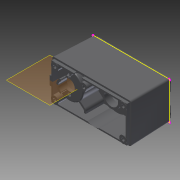
# Autodesk Inventor part: 276-2181-002 Rev1
Saved by Autodesk Inventor 2013 (Build 170138000, 138)
## iProperties
Category: Motors
Company: Autodesk Inc.
Created: 2012-01-21
Part Number: 276-2181-002 Rev1
Material: Generic
Document SubType Name: Modeling
Designer: Autodesk Inc.
Density: 1 g/cm^3
Catalog Web Link: http://www.vexrobotics.com/276-2181.html
Vendor: VEX
Author: Autodesk Inc.
Autodesk Inventor part; units mm, degrees
sketch "Sketch1" plane through (0, 0, 0) normal (0, 0, 1) x (1, 0, 0)
  line L0 (-20, -10) -> (20, -10)
  line L1 (20, -10) -> (20, 10)
  line L2 (-20, 10) -> (20, 10)
  line L3 (-20, -10) -> (-20, 10)
  point P0 (-19.0003, -10)
  point P1 (19.0003, -10)
  point P2 (20, -9.0003)
  point P3 (20, 9.0003)
  point P4 (19.0003, 10)
  point P5 (-19.0003, 10)
  point P6 (-20, 9.0003)
  point P7 (-20, -9.0003)
  constraints: 8 end point, 8 point on line, 1 parallel
extrude "Extrusion1" add sketch "Sketch1" against normal blind 19.9898 draft -1.5
fillet "Fillet3" radius 1.0033 4 edges at (19.7383, 9.7383, -9.9949) (19.7383, -9.7383, -9.9949) (-19.7383, 9.7383, -9.9949) (-19.7383, -9.7383, -9.9949)
sketch "Sketch2" plane through (0, 0, 0) normal (0, 0, 1) x (1, 0, 0)
  arc A0 (-10.02, 6.9107) -> (-9.998, 7.0969) centre (-10.798, 7.0969) ccw
  arc A1 (-10.02, 6.9107) -> (-9.9362, 6.8636) centre (-9.9713, 6.8991) ccw
  arc A2 (-9.0524, 7.5864) -> (-9.9362, 6.8636) centre (-5.7003, 2.586) ccw
  arc A3 (-8.5705, 8.418) -> (-9.0524, 7.5864) centre (-8.188, 7.6409) ccw
  arc A4 (-7.7003, 8.7706) -> (-8.5705, 8.418) centre (-5.7003, 2.586) ccw
  line L0 (-7.7003, 8.7706) -> (-7.7003, 9.2)
  line L1 (-17.3, 9.2) -> (-7.7003, 9.2)
  line L2 (-18.5, 8.5) -> (-9.998, 8.5)
  line L3 (-9.998, 8.5) -> (-9.998, 7.0969)
  line L4 (17.3, -9.2) -> (-17.3, -9.2)
  line L5 (19.2, 7.3) -> (19.2, -7.3)
  line L6 (18.5, -8.5) -> (18.5, 8.5)
  line L7 (-18.5, -8.5) -> (-1.0407, -8.5)
  line L8 (-18.5, 8.5) -> (-18.5, -8.5)
  line L9 (-19.2, 2.3) -> (-19.2, 7.3)
  line L10 (-20, 2.3) -> (-19.2, 2.3)
  line L11 (-20, -2.3) -> (-20, 2.3)
  line L12 (-19.2, -2.3) -> (-20, -2.3)
  line L13 (-19.2, -7.3) -> (-19.2, -2.3)
  line L14 (-17.3, -9.2) -> (-19.0003, -9.2)
  spline S0 degree 3 poles (-19.0003, -9.2) (-19.017, -9.2) (-19.0534, -9.1953) (-19.1011, -9.1753) (-19.1432, -9.1432) (-19.1753, -9.1011) (-19.1953, -9.0534) (-19.2, -9.017) (-19.2, -9.0003) knots -0.917613 -0.917613 -0.917613 -0.917613 -0.780175 -0.642783 -0.505417 -0.368051 -0.230659 -0.093221 -0.093221 -0.093221 -0.093221
  line L15 (-19.2, -9.0003) -> (-19.2, -7.3)
  line L16 (19.0003, -9.2) -> (17.3, -9.2)
  line L17 (19.2, -7.3) -> (19.2, -9.0003)
  spline S1 degree 3 poles (19.2, -9.0003) (19.2, -9.017) (19.1953, -9.0534) (19.1753, -9.1011) (19.1432, -9.1432) (19.1011, -9.1753) (19.0534, -9.1953) (19.017, -9.2) (19.0003, -9.2) knots -0.917613 -0.917613 -0.917613 -0.917613 -0.780175 -0.642783 -0.505417 -0.368051 -0.230659 -0.093221 -0.093221 -0.093221 -0.093221
  line L18 (19.2, 9.0003) -> (19.2, 7.3)
  spline S2 degree 3 poles (19.0003, 9.2) (19.017, 9.2) (19.0534, 9.1953) (19.1011, 9.1753) (19.1432, 9.1432) (19.1753, 9.1011) (19.1953, 9.0534) (19.2, 9.017) (19.2, 9.0003) knots -0.917613 -0.917613 -0.917613 -0.917613 -0.780175 -0.642783 -0.505417 -0.368051 -0.230659 -0.093221 -0.093221 -0.093221 -0.093221
  line L19 (17.3, 9.2) -> (19.0003, 9.2)
  line L20 (-3.7003, 9.2) -> (17.3, 9.2)
  line L21 (-3.7003, 8.7706) -> (-3.7003, 9.2)
  arc A5 (-3.0033, 8.5) -> (-3.7003, 8.7706) centre (-5.7003, 2.586) ccw
  line L22 (18.5, 8.5) -> (-3.0033, 8.5)
  arc A6 (-1.0407, -8.5) -> (5.3473, -8.5) centre (2.1533, -1.4937) ccw
  line L23 (5.3473, -8.5) -> (18.5, -8.5)
  line L24 (-9.998, 8.5) -> (-15.8269, 8.5)
  line L25 (-9.998, 7.0969) -> (-9.998, 8.5)
  arc A7 (-10.02, 6.9107) -> (-9.998, 7.0969) centre (-10.798, 7.0969) ccw
  arc A8 (-10.02, 6.9107) -> (-9.9362, 6.8636) centre (-9.9713, 6.8991) ccw
  arc A9 (-9.0524, 7.5864) -> (-9.9362, 6.8636) centre (-5.7003, 2.586) ccw
  arc A10 (-8.5705, 8.418) -> (-9.0524, 7.5864) centre (-8.188, 7.6409) ccw
  arc A11 (-7.7003, 8.7706) -> (-8.5705, 8.418) centre (-5.7003, 2.586) ccw
  line L26 (-7.7003, 9.2) -> (-7.7003, 8.7706)
  line L27 (-17.3, 9.2) -> (-7.7003, 9.2)
  line L28 (-19.0003, 9.2) -> (-17.3, 9.2)
  spline S3 degree 3 poles (-19.2, 9.0003) (-19.2, 9.017) (-19.1953, 9.0534) (-19.1753, 9.1011) (-19.1432, 9.1432) (-19.1011, 9.1753) (-19.0534, 9.1953) (-19.017, 9.2) (-19.0003, 9.2) knots -0.917613 -0.917613 -0.917613 -0.917613 -0.780175 -0.642783 -0.505417 -0.368051 -0.230659 -0.093221 -0.093221 -0.093221 -0.093221
  line L29 (-19.2, 7.3) -> (-19.2, 9.0003)
  line L30 (-1.0407, -8.5) -> (5.3473, -8.5)
  point P0 (0, 0)
  point P1 (0, 0)
  constraints: 62 end point, 24 point on circle, 12 centre point, 1 perpendicular, 1 point on line, 8 other
extrude "Extrusion2" add sketch "Sketch2" along normal blind 1.2954
sketch "Sketch4" plane through (0, 0, 0) normal (0, 0, 1) x (1, 0, 0)
  line L0 (-7.7003, 9.2) -> (-7.7003, 8.7706) projected
  arc A0 (-7.7003, 8.7706) -> (-8.5705, 8.418) centre (-5.7003, 2.586) ccw projected
  arc A1 (-8.5705, 8.418) -> (-9.0524, 7.5864) centre (-8.188, 7.6409) ccw projected
  arc A2 (-9.0524, 7.5864) -> (-9.9362, 6.8636) centre (-5.7003, 2.586) ccw projected
  arc A3 (-10.02, 6.9107) -> (-9.9362, 6.8636) centre (-9.9713, 6.8991) ccw projected
  arc A4 (-10.02, 6.9107) -> (-9.998, 7.0969) centre (-10.798, 7.0969) ccw projected
  line L1 (-9.998, 7.0969) -> (-9.998, 8.5) projected
  line L2 (-9.998, 8.5) -> (-18.5, 8.5) projected
  line L3 (-18.5, 8.5) -> (-18.5, -8.5) projected
  line L4 (-18.5, -8.5) -> (18.5, -8.5) projected
  line L5 (18.5, -8.5) -> (18.5, 8.5) projected
  line L6 (18.5, 8.5) -> (-3.0033, 8.5) projected
  arc A5 (-3.0033, 8.5) -> (-3.7003, 8.7706) centre (-5.7003, 2.586) ccw projected
  arc A6 (-3.0033, 8.5) -> (-7.7003, 8.7706) centre (-5.7003, 2.586) ccw
  point P0 (0, 0)
  constraints: 3 point on circle, 2 end point, 1 centre point, 1 coincident
extrude "Extrusion3" cut sketch "Sketch4" against normal blind 10.6934
sketch "Sketch5" plane through (0, 0, 1.2954) normal (0, 0, 1) x (1, 0, 0)
  line L0 (-18.5, -8.5) -> (18.5, -8.5) projected
  line L1 (-18.5, 8.5) -> (-18.5, -8.5) projected
  line L2 (-9.998, 8.5) -> (-18.5, 8.5) projected
  line L3 (-9.998, 7.0969) -> (-9.998, 8.5) projected
  arc A0 (-10.02, 6.9107) -> (-9.998, 7.0969) centre (-10.798, 7.0969) ccw projected
  arc A1 (-10.02, 6.9107) -> (-9.9362, 6.8636) centre (-9.9713, 6.8991) ccw projected
  arc A2 (-9.0524, 7.5864) -> (-9.9362, 6.8636) centre (-5.7003, 2.586) ccw projected
  arc A3 (-8.5705, 8.418) -> (-9.0524, 7.5864) centre (-8.188, 7.6409) ccw projected
  arc A4 (-7.7003, 8.7706) -> (-8.5705, 8.418) centre (-5.7003, 2.586) ccw projected
  line L4 (-7.7003, 9.2) -> (-7.7003, 8.7706) projected
  line L5 (-19.0003, 9.2) -> (-7.7003, 9.2) projected
  line L6 (-19.2, 2.3) -> (-19.2, 9.0003) projected
  line L7 (-20, 2.3) -> (-19.2, 2.3) projected
  line L8 (-20, -2.3) -> (-20, 2.3) projected
  line L9 (-19.2, -2.3) -> (-20, -2.3) projected
  line L10 (-19.2, -9.0003) -> (-19.2, -2.3) projected
  line L11 (19.0003, -9.2) -> (-19.0003, -9.2) projected
  line L12 (19.2, 9.0003) -> (19.2, -9.0003) projected
  line L13 (-3.7003, 9.2) -> (19.0003, 9.2) projected
  line L14 (-3.7003, 8.7706) -> (-3.7003, 9.2) projected
  arc A5 (-3.0033, 8.5) -> (-3.7003, 8.7706) centre (-5.7003, 2.586) ccw projected
  line L15 (18.5, 8.5) -> (-3.0033, 8.5) projected
  line L16 (18.5, -8.5) -> (18.5, 8.5) projected
  point P0 (0, 0)
  constraints: 4 other
sketch "Sketch6" plane through (0, 0, 1.2954) normal (0, 0, 1) x (1, 0, 0)
  line L0 (-18.5, -8.5) -> (18.5, -8.5) projected
  arc A0 (-1.0407, -8.5) -> (5.3473, -8.5) centre (2.1533, -1.4937) ccw projected
  point P0 (0, 0)
extrude "Extrusion4" cut sketch "Sketch6" against normal up to surface (11.9888 mm away)
sketch "Sketch8" plane through (0, 0, -19.9898) normal (0, 0, -1) x (-1, 0, 0)
  line L0 (16.9263, -8.6763) -> (-16.9263, -8.6763)
  line L1 (17.9763, -7.9763) -> (-15.5263, -7.9763)
  spline S0 degree 3 poles (-18.6763, 8.4766) (-18.6763, 8.4933) (-18.6716, 8.5297) (-18.6516, 8.5774) (-18.6195, 8.6195) (-18.5774, 8.6516) (-18.5297, 8.6716) (-18.4933, 8.6763) (-18.4766, 8.6763) knots -0.917613 -0.917613 -0.917613 -0.917613 -0.780175 -0.642783 -0.505417 -0.368052 -0.230659 -0.093221 -0.093221 -0.093221 -0.093221
  line L2 (-18.4766, 8.6763) -> (-16.9263, 8.6763)
  line L3 (-16.9263, 8.6763) -> (16.9263, 8.6763)
  line L4 (18.6763, 8.4766) -> (18.6763, 6.9263)
  spline S1 degree 3 poles (18.4766, 8.6763) (18.4933, 8.6763) (18.5297, 8.6716) (18.5774, 8.6516) (18.6195, 8.6195) (18.6516, 8.5774) (18.6716, 8.5297) (18.6763, 8.4933) (18.6763, 8.4766) knots -0.917613 -0.917613 -0.917613 -0.917613 -0.780175 -0.642783 -0.505417 -0.368052 -0.230659 -0.093221 -0.093221 -0.093221 -0.093221
  line L5 (16.9263, 8.6763) -> (18.4766, 8.6763)
  line L6 (17.9763, 7.9763) -> (-17.9763, 7.9763)
  line L7 (-18.6763, 3) -> (-18.6763, 6.9263)
  line L8 (-18.0037, 3) -> (-18.6763, 3)
  arc A0 (-17.9763, 3.0621) -> (-18.0037, 3) centre (-11.1298, 0) ccw
  line L9 (-17.9763, 7.9763) -> (-17.9763, 3.0621)
  line L10 (-18.6763, 6.9263) -> (-18.6763, 8.4766)
  line L11 (18.6763, 6.9263) -> (18.6763, -6.9263)
  line L12 (18.4766, -8.6763) -> (16.9263, -8.6763)
  spline S2 degree 3 poles (18.6763, -8.4766) (18.6763, -8.4933) (18.6716, -8.5297) (18.6516, -8.5774) (18.6195, -8.6195) (18.5774, -8.6516) (18.5297, -8.6716) (18.4933, -8.6763) (18.4766, -8.6763) knots -0.917613 -0.917613 -0.917613 -0.917613 -0.780175 -0.642783 -0.505417 -0.368052 -0.230659 -0.093221 -0.093221 -0.093221 -0.093221
  line L13 (18.6763, -6.9263) -> (18.6763, -8.4766)
  line L14 (17.9763, -7.9763) -> (17.9763, 7.9763)
  line L15 (16.9263, -8.6763) -> (-16.9263, -8.6763)
  line L16 (-17.9763, -7.9763) -> (15.5263, -7.9763)
  line L17 (-16.9263, -8.6763) -> (-18.4766, -8.6763)
  spline S3 degree 3 poles (-18.4766, -8.6763) (-18.4933, -8.6763) (-18.5297, -8.6716) (-18.5774, -8.6516) (-18.6195, -8.6195) (-18.6516, -8.5774) (-18.6716, -8.5297) (-18.6763, -8.4933) (-18.6763, -8.4766) knots -0.917613 -0.917613 -0.917613 -0.917613 -0.780175 -0.642783 -0.505417 -0.368052 -0.230659 -0.093221 -0.093221 -0.093221 -0.093221
  line L18 (-18.6763, -8.4766) -> (-18.6763, -6.9263)
  line L19 (-18.6763, -6.9263) -> (-18.6763, -3)
  line L20 (-18.6763, -3) -> (-18.0037, -3)
  arc A1 (-18.0037, -3) -> (-17.9763, -3.0621) centre (-11.1298, 0) ccw
  line L21 (-17.9763, -3.0621) -> (-17.9763, -7.9763)
  point P0 (0, 0)
  point P1 (0, 0)
  constraints: 44 end point, 4 point on circle, 2 centre point, 2 point on line, 8 other
extrude "Extrusion5" add sketch "Sketch8" along normal blind 1.2954
sketch "Sketch9" plane through (0, 0, -19.9898) normal (0, 0, -1) x (-1, 0, 0)
  line L0 (-18.6763, -3) -> (-18.0037, -3) projected
  line L1 (-17.9763, -3.0621) -> (-17.9763, -7.9763) projected
  line L2 (-17.9763, -7.9763) -> (17.9763, -7.9763) projected
  line L3 (17.9763, -7.9763) -> (17.9763, 7.9763) projected
  line L4 (17.9763, 7.9763) -> (-17.9763, 7.9763) projected
  line L5 (-17.9763, 7.9763) -> (-17.9763, 3.0621) projected
  arc A0 (-17.9763, 3.0621) -> (-18.0037, 3) centre (-11.1298, 0) ccw projected
  line L6 (-18.0037, 3) -> (-18.6763, 3) projected
  line L7 (-19.4765, -9.4765) -> (-19.4765, 9.4765) projected
  arc A1 (-17.9763, 3.0621) -> (-17.9763, -3.0621) centre (-11.1298, 0) ccw
  line L8 (-17.9763, 3.0621) -> (-17.9763, 3)
  line L9 (-17.9763, -3) -> (-17.9763, -3.0621)
  point P0 (-19.4765, 9.0003)
  point P1 (-19.4765, -9.0003)
  point P2 (0, 0)
  constraints: 4 end point, 2 parallel, 2 point on circle, 2 point on line, 1 centre point, 1 coincident, 1 concentric
extrude "Extrusion6" cut sketch "Sketch9" against normal blind 9.0932
ref_plane "Work Plane1" through (0, 0, -21.4884) normal (0, 0, -1) x (-1, 0, 0)
sketch "Sketch10" plane through (0, 0, -21.4884) normal (0, 0, -1) x (-1, 0, 0)
  arc A0 (15.5263, -7.9763) -> (16.9263, -8.6763) centre (16.9263, -6.9263) ccw
  arc A1 (-16.9263, -8.6763) -> (-15.5263, -7.9763) centre (-16.9263, -6.9263) ccw
  circle A2 centre (-16.9263, -6.9263) radius 0.8
  circle A3 centre (-16.9263, 6.9263) radius 0.8
  circle A4 centre (16.9263, 6.9263) radius 0.8
  circle A5 centre (16.9263, -6.9263) radius 0.8
  arc A6 (18.6763, 6.9263) -> (16.9263, 8.6763) centre (16.9263, 6.9263) ccw
  arc A7 (16.9263, 8.6763) -> (15.5263, 7.9763) centre (16.9263, 6.9263) ccw
  arc A8 (-15.5263, 7.9763) -> (-16.9263, 8.6763) centre (-16.9263, 6.9263) ccw
  arc A9 (-16.9263, 8.6763) -> (-18.6763, 6.9263) centre (-16.9263, 6.9263) ccw
  arc A10 (-17.9763, 5.5263) -> (-15.5263, 7.9763) centre (-16.9263, 6.9263) ccw
  arc A11 (17.9763, 5.5263) -> (18.6763, 6.9263) centre (16.9263, 6.9263) ccw
  arc A12 (15.5263, 7.9763) -> (17.9763, 5.5263) centre (16.9263, 6.9263) ccw
  arc A13 (-18.6763, 6.9263) -> (-17.9763, 5.5263) centre (-16.9263, 6.9263) ccw
  arc A14 (16.9263, -8.6763) -> (18.6763, -6.9263) centre (16.9263, -6.9263) ccw
  arc A15 (18.6763, -6.9263) -> (17.9763, -5.5263) centre (16.9263, -6.9263) ccw
  arc A16 (15.5263, -7.9763) -> (16.9263, -8.6763) centre (16.9263, -6.9263) ccw
  arc A17 (17.9763, -5.5263) -> (15.5263, -7.9763) centre (16.9263, -6.9263) ccw
  arc A18 (-18.6763, -6.9263) -> (-16.9263, -8.6763) centre (-16.9263, -6.9263) ccw
  arc A19 (-17.9763, -5.5263) -> (-18.6763, -6.9263) centre (-16.9263, -6.9263) ccw
  arc A20 (-15.5263, -7.9763) -> (-17.9763, -5.5263) centre (-16.9263, -6.9263) ccw
  arc A21 (-16.9263, -8.6763) -> (-15.5263, -7.9763) centre (-16.9263, -6.9263) ccw
  point P0 (0, 0)
  point P1 (0, 0)
  constraints: 36 point on circle, 22 centre point
extrude "Extrusion7" add sketch "Sketch10" against normal up to surface (10.5918 mm away)
ref_plane "Work Plane2" through (0, 0, 1.4986) normal (0, 0, 1) x (1, 0, 0)
ref_plane "Work Plane3" through (0, 0, -1.5046) normal (0, 0, 1) x (1, 0, 0)
sketch "Sketch12" plane through (0, 0, -1.5046) normal (0, 0, 1) x (1, 0, 0)
  arc A0 (-9.9362, 6.8636) -> (-9.9051, 7.0969) centre (-10.798, 7.0969) ccw
  arc A1 (-9.9362, 6.8636) -> (-9.9362, 6.8636) centre (-9.9713, 6.8991) ccw
  arc A2 (-17.3, -9.2) -> (-15.8269, -8.5) centre (-17.3, -7.3) ccw
  line L0 (-18.5, 4.2) -> (-18.5, -4.2)
  arc A3 (-19.2, 7.3) -> (-18.5, 5.8269) centre (-17.3, 7.3) ccw
  line L1 (-19.2, 2.3) -> (-19.2, 7.3)
  line L2 (-20, 2.3) -> (-19.2, 2.3)
  line L3 (-20, -2.3) -> (-20, 2.3)
  line L4 (-19.2, -2.3) -> (-20, -2.3)
  line L5 (-19.2, -7.3) -> (-19.2, -2.3)
  arc A4 (-19.2, -7.3) -> (-17.3, -9.2) centre (-17.3, -7.3) ccw
  line L6 (-17.3, -9.2) -> (-19.0003, -9.2)
  spline S0 degree 3 poles (-19.0003, -9.2) (-19.017, -9.2) (-19.0534, -9.1953) (-19.1011, -9.1753) (-19.1432, -9.1432) (-19.1753, -9.1011) (-19.1953, -9.0534) (-19.2, -9.017) (-19.2, -9.0003) knots -0.917613 -0.917613 -0.917613 -0.917613 -0.780175 -0.642783 -0.505417 -0.368051 -0.230659 -0.093221 -0.093221 -0.093221 -0.093221
  line L7 (-19.2, -9.0003) -> (-19.2, -7.3)
  arc A5 (-18.5, -5.8269) -> (-19.2, -7.3) centre (-17.3, -7.3) ccw
  line L8 (-3.7003, 8.7706) -> (-3.7003, 9.2)
  arc A6 (-9.9362, 6.8636) -> (-9.9051, 7.0969) centre (-10.798, 7.0969) ccw
  arc A7 (-9.9362, 6.8636) -> (-9.9362, 6.8636) centre (-9.9713, 6.8991) ccw
  spline S1 degree 3 poles (-19.2, 9.0003) (-19.2, 9.017) (-19.1953, 9.0534) (-19.1753, 9.1011) (-19.1432, 9.1432) (-19.1011, 9.1753) (-19.0534, 9.1953) (-19.017, 9.2) (-19.0003, 9.2) knots -0.917613 -0.917613 -0.917613 -0.917613 -0.780175 -0.642783 -0.505417 -0.368051 -0.230659 -0.093221 -0.093221 -0.093221 -0.093221
  line L9 (-19.2, 7.3) -> (-19.2, 9.0003)
  arc A8 (-7.3, -4.2) -> (-18.5, 4.2) centre (-12.9, 0) ccw
  arc A9 (-17.3533, 5.4007) -> (-18.4825, 4.2232) centre (-12.9, 0) ccw
  arc A10 (-7.3, 4.2) -> (-9.3472, 6.0314) centre (-12.9, 0) ccw
  arc A11 (-9.1281, -5.8969) -> (-8.0571, -5.0543) centre (-12.9, 0) ccw
  arc A12 (-18.5, -4.2) -> (-7.3, -4.2) centre (-12.9, 0) ccw
  arc A13 (-18.4825, -4.2232) -> (-17.3533, -5.4007) centre (-12.9, 0) ccw
  line L10 (-20, -8.997) -> (-20, -2.3) projected
  circle A14 centre (-17.3, -7.3) radius 0.8 projected
  point P0 (-20, 2.3)
  point P1 (-20, 9.0003)
  point P2 (-20, -9.0003)
  point P3 (-20, -10)
  constraints: 30 point on circle, 20 end point, 14 centre point, 4 other
sketch "Sketch11" plane through (0, 0, 1.4986) normal (0, 0, 1) x (1, 0, 0)
  arc A0 (-15.8269, 8.5) -> (-17.3, 9.2) centre (-17.3, 7.3) ccw
  arc A1 (-17.3, -9.2) -> (-15.8269, -8.5) centre (-17.3, -7.3) ccw
  arc A2 (17.3, -9.2) -> (19.2, -7.3) centre (17.3, -7.3) ccw
  arc A3 (19.2, 7.3) -> (17.3, 9.2) centre (17.3, 7.3) ccw
  arc A4 (17.3, 9.2) -> (15.8269, 8.5) centre (17.3, 7.3) ccw
  arc A5 (15.8269, 8.5) -> (18.5, 5.8269) centre (17.3, 7.3) ccw
  arc A6 (19.2, -7.3) -> (18.5, -5.8269) centre (17.3, -7.3) ccw
  arc A7 (-15.8269, -8.5) -> (-18.5, -5.8269) centre (-17.3, -7.3) ccw
  arc A8 (-19.2, 7.3) -> (-18.5, 5.8269) centre (-17.3, 7.3) ccw
  arc A9 (-19.2, -7.3) -> (-17.3, -9.2) centre (-17.3, -7.3) ccw
  arc A10 (-18.5, -5.8269) -> (-19.2, -7.3) centre (-17.3, -7.3) ccw
  arc A11 (15.8269, -8.5) -> (17.3, -9.2) centre (17.3, -7.3) ccw
  arc A12 (18.5, -5.8269) -> (15.8269, -8.5) centre (17.3, -7.3) ccw
  arc A13 (18.5, 5.8269) -> (19.2, 7.3) centre (17.3, 7.3) ccw
  arc A14 (-18.5, 5.8269) -> (-15.8269, 8.5) centre (-17.3, 7.3) ccw
  arc A15 (-17.3, 9.2) -> (-19.2, 7.3) centre (-17.3, 7.3) ccw
  arc A16 (-15.8269, 8.5) -> (-17.3, 9.2) centre (-17.3, 7.3) ccw
  circle A17 centre (-17.3, 7.3) radius 0.8
  circle A18 centre (17.3, 7.3) radius 0.8
  circle A19 centre (17.3, -7.3) radius 0.8
  circle A20 centre (-17.3, -7.3) radius 0.8
  point P0 (0, 0)
  point P1 (0, 0)
  constraints: 34 point on circle, 21 centre point
extrude "Extrusion10" add sketch "Sketch12" against normal up to surface (9.1888 mm away) contours A8 A12 A11 L0
fillet "Fillet2" radius 0.508 1 edges at (-5.9, 0, -1.5046)
extrude "Extrusion11" add sketch "Sketch11" against normal up to surface (12.192 mm away)
sketch "Sketch13" plane through (0, 0, -1.5046) normal (0, 0, 1) x (1, 0, 0)
  arc A0 (-10.02, 6.9107) -> (-9.998, 7.0969) centre (-10.798, 7.0969) ccw
  arc A1 (-10.02, 6.9107) -> (-9.9362, 6.8636) centre (-9.9713, 6.8991) ccw
  arc A2 (-9.0524, 7.5864) -> (-9.9362, 6.8636) centre (-5.7003, 2.586) ccw
  arc A3 (-8.5705, 8.418) -> (-9.0524, 7.5864) centre (-8.188, 7.6409) ccw
  arc A4 (-7.7003, 8.7706) -> (-8.5705, 8.418) centre (-5.7003, 2.586) ccw
  line L0 (-7.7003, 8.7706) -> (-7.7003, 9.2)
  line L1 (-17.3, 9.2) -> (-7.7003, 9.2)
  arc A5 (-15.8269, 8.5) -> (-17.3, 9.2) centre (-17.3, 7.3) ccw
  line L2 (-15.8269, 8.5) -> (-9.998, 8.5)
  line L3 (-9.998, 8.5) -> (-9.998, 7.0969)
  arc A6 (-13.1914, 6.9939) -> (-15.5957, 6.4601) centre (-12.9, 0) ccw
  arc A7 (-17.3533, 5.4007) -> (-18.4825, 4.2232) centre (-12.9, 0) ccw
  arc A8 (-7.3, 4.2) -> (-9.3472, 6.0314) centre (-12.9, 0) ccw
  line L4 (-6.9, 0.9857) -> (-6.9, -3)
  arc A9 (-7.3, -4.2) -> (-6.9, -3) centre (-8.9, -3) ccw
  arc A10 (-9.1281, -5.8969) -> (-8.0571, -5.0543) centre (-12.9, 0) ccw
  arc A11 (-15.5957, -6.4601) -> (-10.5533, -6.5949) centre (-12.9, 0) ccw
  arc A12 (-18.4825, -4.2232) -> (-17.3533, -5.4007) centre (-12.9, 0) ccw
  circle A13 centre (-12.9, 4.25) radius 0.8
  arc A14 (-10.4616, 6.2698) -> (-10.9451, 5.541) centre (-5.7003, 2.586) ccw
  arc A15 (-10.4616, 6.2698) -> (-10.5186, 6.3472) centre (-10.5011, 6.3004) ccw
  arc A16 (-10.798, 6.2969) -> (-10.5186, 6.3472) centre (-10.798, 7.0969) ccw
  line L5 (-10.798, 6.2969) -> (-11.6593, 6.2969)
  arc A17 (-11.6593, 6.2969) -> (-11.8164, 6.0319) centre (-5.7003, 2.586) ccw
  arc A18 (-11.8164, 6.0319) -> (-10.9451, 5.541) centre (-11.3807, 5.7865) ccw
  arc A19 (-9.7096, 5.6632) -> (-9.0359, 7.4642) centre (-10.798, 7.0969) ccw
  arc A20 (-14.4318, 2.2839) -> (-14.4318, -2.2839) centre (-12.9, 0) ccw
  arc A21 (-14.4318, 2.2839) -> (-14.9888, 3.1144) centre (-14.7103, 2.6991) ccw
  arc A22 (-14.9888, 3.1144) -> (-14.9888, -3.1144) centre (-12.9, 0) ccw
  arc A23 (-14.9888, -3.1144) -> (-14.4318, -2.2839) centre (-14.7103, -2.6991) ccw
  circle A24 centre (-12.9, -4.25) radius 0.8
  arc A25 (-9.0524, 7.5864) -> (-9.0359, 7.4642) centre (-8.188, 7.6409) ccw
  arc A26 (-9.0524, 7.5864) -> (-9.9362, 6.8636) centre (-5.7003, 2.586) ccw
  arc A27 (-10.02, 6.9107) -> (-9.9362, 6.8636) centre (-9.9713, 6.8991) ccw
  arc A28 (-10.5186, 6.3472) -> (-10.02, 6.9107) centre (-10.798, 7.0969) ccw
  arc A29 (-10.4616, 6.2698) -> (-10.5186, 6.3472) centre (-10.5011, 6.3004) ccw
  arc A30 (-10.4616, 6.2698) -> (-10.9451, 5.541) centre (-5.7003, 2.586) ccw
  arc A31 (-11.8164, 6.0319) -> (-10.9451, 5.541) centre (-11.3807, 5.7865) ccw
  arc A32 (-11.6593, 6.2969) -> (-11.8164, 6.0319) centre (-5.7003, 2.586) ccw
  line L6 (-12.398, 6.2969) -> (-11.6593, 6.2969)
  arc A33 (-12.9307, 6.5) -> (-12.398, 6.2969) centre (-12.398, 7.0969) ccw
  spline S0 degree 3 poles (-12.9307, 6.5) (-13.2056, 6.4986) (-13.4818, 6.4798) (-13.7538, 6.4438) (-14.0937, 6.3989) (-14.429, 6.327) (-14.7597, 6.2283) (-14.8259, 6.2085) (-14.8947, 6.1868) (-14.962, 6.1643) (-15.3657, 6.0294) (-15.7526, 5.8563) (-16.1226, 5.6449) (-16.3693, 5.5041) (-16.6067, 5.3472) (-16.8317, 5.1763) (-17.0568, 5.0054) (-17.2704, 4.8199) (-17.4726, 4.6197) (-17.5737, 4.5196) (-17.6671, 4.4208) (-17.7584, 4.3182) (-18.0321, 4.0105) (-18.275, 3.6784) (-18.4869, 3.3221) knots 0.474807 0.474807 0.474807 0.474807 0.540456 0.540456 0.540456 0.622517 0.622517 0.622517 0.638929 0.638929 0.638929 0.737403 0.737403 0.737403 0.803052 0.803052 0.803052 0.868702 0.868702 0.868702 0.901526 0.901526 0.901526 1 1 1 1
  line L7 (-18.4869, 3.3221) -> (-18.4869, -3.3221)
  spline S1 degree 3 poles (-18.4869, -3.3221) (-18.2719, -3.6837) (-18.0245, -4.0207) (-17.745, -4.3332) (-17.705, -4.3778) (-17.6655, -4.4208) (-17.6232, -4.4656) (-17.2847, -4.8236) (-16.9095, -5.1397) (-16.4993, -5.4125) (-16.1403, -5.6512) (-15.7616, -5.8521) (-15.3633, -6.0152) (-15.3064, -6.0385) (-15.2475, -6.0616) (-15.1913, -6.0827) (-14.7419, -6.252) (-14.2784, -6.3703) (-13.8028, -6.437) (-13.3867, -6.4954) (-12.9691, -6.5132) (-12.5501, -6.4906) (-12.4902, -6.4873) (-12.4318, -6.4834) (-12.3704, -6.4784) (-11.8793, -6.4383) (-11.3981, -6.3432) (-10.9286, -6.1938) (-10.5178, -6.0631) (-10.1242, -5.8933) (-9.7478, -5.6845) (-9.694, -5.6546) (-9.6391, -5.6232) (-9.5875, -5.5926) (-9.1744, -5.348) (-8.7927, -5.0608) (-8.4426, -4.7309) knots 0 0 0 0 0.109375 0.109375 0.109375 0.125 0.125 0.125 0.25 0.25 0.25 0.359375 0.359375 0.359375 0.375 0.375 0.375 0.5 0.5 0.5 0.609375 0.609375 0.609375 0.625 0.625 0.625 0.75 0.75 0.75 0.859375 0.859375 0.859375 0.875 0.875 0.875 1 1 1 1
  line L8 (-8.4426, -4.7309) -> (-5.8572, -6.9003)
  arc A34 (-5.5, -7.6663) -> (-5.8572, -6.9003) centre (-6.5, -7.6663) ccw
  line L9 (-5.5, -8.4869) -> (-5.5, -7.6663)
  line L10 (-5.5, -8.4869) -> (-4.5, -8.4869)
  line L11 (-4.5, -7.6663) -> (-4.5, -8.4869)
  arc A35 (-4.5, -7.6663) -> (-5.2144, -6.1342) centre (-6.5, -7.6663) ccw
  line L12 (-7.7692, -3.9905) -> (-5.2144, -6.1342)
  line L13 (-7.7692, -3.9905) -> (-7.7, -3.9)
  ellipse E0 centre (-9.0235, -2.959) end of major axis (-7.4764, -3.4727) minor radius 1.5621 (-7.7, -3.9) -> (-7.4, -3) ccw
  line L14 (-7.4, -3) -> (-7.4, 1.5319)
  arc A36 (-7.4, 1.5319) -> (-5.0168, 0.7064) centre (-5.7003, 2.586) ccw
  arc A37 (-3.7695, 3.1075) -> (-5.0168, 0.7064) centre (2.1533, -1.4937) ccw
  arc A38 (-3.7695, 3.1075) -> (-7.4, 1.5319) centre (-5.7003, 2.586) ccw
  arc A39 (-7.4831, 3.4924) -> (-7.7, 3.9) centre (-8.9, 3) ccw
  spline S2 degree 3 poles (-7.7, 3.9) (-7.9674, 4.2565) (-8.2675, 4.5814) (-8.6004, 4.8748) (-8.6836, 4.9481) (-8.7685, 5.0194) (-8.8582, 5.0906) (-8.948, 5.1619) (-9.0393, 5.2306) (-9.1323, 5.2968) (-9.3182, 5.4292) (-9.5107, 5.5513) (-9.7096, 5.6632) knots 0 0 0 0 0.5 0.5 0.5 0.625 0.625 0.625 0.75 0.75 0.75 1 1 1 1
  arc A40 (-9.7096, 5.6632) -> (-9.0359, 7.4642) centre (-10.798, 7.0969) ccw
  circle A41 centre (-12.9, -4.25) radius 0.8
  circle A42 centre (-12.9, 4.25) radius 0.8
  circle A43 centre (-5.7003, 2.586) radius 0.775
  arc A44 (-14.4318, -2.2839) -> (-14.4318, 2.2839) centre (-12.9, 0) ccw
  arc A45 (-14.9888, -3.1144) -> (-14.4318, -2.2839) centre (-14.7103, -2.6991) ccw
  arc A46 (-14.9888, 3.1144) -> (-14.9888, -3.1144) centre (-12.9, 0) ccw
  arc A47 (-14.4318, 2.2839) -> (-14.9888, 3.1144) centre (-14.7103, 2.6991) ccw
  arc A48 (-6.9, 0.9857) -> (-7.1484, 3.9654) centre (-5.7003, 2.586) ccw
  arc A49 (-15.5957, -6.4601) -> (-10.5533, -6.5949) centre (-12.9, 0) ccw
  arc A50 (-15.5957, -6.4601) -> (-15.5957, 6.4601) centre (-12.9, 0) ccw
  arc A51 (-8.4426, -4.7309) -> (-7.7692, -3.9905) centre (-13.069, 0.1537) ccw
  point P0 (0, 0)
  point P1 (17.3, -9.2)
  constraints: 93 point on circle, 51 centre point, 30 end point, 10 other
extrude "Extrusion12" add sketch "Sketch13" along normal up to surface (2.8 mm away) contours A15 A14 A18 A17 L5 A16
extrude "Extrusion13" add sketch "Sketch13" along normal up to surface (2.8 mm away) contours A20 A23 A22 A21
extrude "Extrusion14" add sketch "Sketch13" against normal up to surface (9.1888 mm away) contours A51 L12 A50 L8 | L12 A35 L11 L10 L9 A34 L8 A50
extrude "Extrusion15" add sketch "Sketch13" against normal up to surface (9.1888 mm away) contours A50 A43 A36 A38 | A38 A37 A36 A50 A43 | A48 A37
extrude "Extrusion16" cut sketch "Sketch13" against normal blind 4.9 contours A48 A37
sketch "Sketch14" plane through (0, 0, -10.6934) normal (0, 0, 1) x (1, 0, 0)
  circle A0 centre (2.1533, -1.4937) radius 4.5
  circle A1 centre (2.1533, -1.4937) radius 3.5
  arc A2 (8.9398, -0.5) -> (8.9398, 0.5) centre (10.8763, 0) ccw
  line L0 (6.1875, 0.5) -> (8.9398, 0.5)
  arc A3 (6.5422, -0.5) -> (6.1875, 0.5) centre (2.1533, -1.4937) ccw
  line L1 (8.9398, -0.5) -> (6.5422, -0.5)
  circle A4 centre (10.8763, 0) radius 0.775
  circle A5 centre (2.1533, -1.4937) radius 4.5
  circle A6 centre (2.1533, -1.4937) radius 3.5
  arc A7 (8.9398, -0.5) -> (8.9398, 0.5) centre (10.8763, 0) ccw
  line L2 (6.1875, 0.5) -> (8.9398, 0.5)
  arc A8 (6.5422, -0.5) -> (6.1875, 0.5) centre (2.1533, -1.4937) ccw
  line L3 (8.9398, -0.5) -> (6.5422, -0.5)
  circle A9 centre (10.8763, 0) radius 0.775
  ellipse E0 centre (18.9997, 8.9997) end of major axis (19.7072, 9.7072) minor radius 1 (20, 9.0003) -> (19.0003, 10) ccw
  ellipse E1 centre (18.9997, 8.9997) end of major axis (18.2921, 8.2921) minor radius 1 (20, 9.0003) -> (19.0003, 10) ccw projected
  point P0 (0, 0)
  point P1 (0, 0)
  point P2 (0, 0)
  constraints: 10 centre point, 8 end point, 8 point on circle, 5 other
extrude "Extrusion17" add sketch "Sketch14" along normal blind 3 contours A0
extrude "Extrusion18" add sketch "Sketch14" along normal blind 2.9 contours A0 L0 A2 L1
sketch "Sketch15" plane through (0, 0, -10.8966) normal (0, 0, -1) x (-1, 0, 0)
  arc A0 (12.4899, 6.4015) -> (12.4899, 7.9763) centre (12.4899, 7.1889) ccw
  line L0 (12.4899, 6.4015) -> (10.8897, 6.4015)
  arc A1 (10.8897, 7.9763) -> (10.8897, 6.4015) centre (10.8897, 7.1889) ccw
  arc A2 (-17.8969, 5.4701) -> (-15.4701, 7.8969) centre (-16.9263, 6.9263) ccw
  line L1 (-17.8969, 5.4701) -> (-17.8969, 3.2338)
  arc A3 (-17.8969, 3.2338) -> (-17.8969, -3.2338) centre (-11.1298, 0) ccw
  line L2 (-17.8969, -5.4701) -> (-17.8969, -3.2338)
  arc A4 (-15.4701, -7.8969) -> (-17.8969, -5.4701) centre (-16.9263, -6.9263) ccw
  arc A5 (8, -5.9763) -> (8, -7.9763) centre (8, -6.9763) ccw
  line L3 (8, -5.9763) -> (9.6, -5.9763)
  arc A6 (9.6, -7.9763) -> (9.6, -5.9763) centre (9.6, -6.9763) ccw
  arc A7 (17.8969, -5.4701) -> (15.4701, -7.8969) centre (16.9263, -6.9263) ccw
  arc A8 (7.8311, -3.3373) -> (17.9763, -3.3262) centre (12.9, 0) ccw
  line L4 (7.8311, -3.3373) -> (7.8311, 3.3373)
  arc A9 (17.9763, 3.3262) -> (7.8311, 3.3373) centre (12.9, 0) ccw
  arc A10 (15.4701, 7.8969) -> (17.8969, 5.4701) centre (16.9263, 6.9263) ccw
  circle A11 centre (-11.1298, 0) radius 3.5
  circle A12 centre (-2.1533, -1.4937) radius 3.5
  line L5 (17.9763, -5.5263) -> (17.9763, 5.5263) projected
  line L6 (17.9763, 3.3262) -> (17.9763, -3.3262)
  line L7 (10.8897, 7.9763) -> (12.4899, 7.9763)
  line L8 (15.5263, 7.9763) -> (-15.5263, 7.9763) projected
  circle A13 centre (-11.1298, 0) radius 2.5019
  line L9 (8, -7.9763) -> (9.6, -7.9763)
  line L10 (-15.5263, -7.9763) -> (15.5263, -7.9763) projected
  point P0 (0, 0)
  point P1 (15.4701, -7.8969)
  dimension "d45" = 0.7874
  dimension "d46" = 5.4864
  dimension "d47" = 1.6002
  dimension "d50" = 5.0038
  dimension "d55" = 8.3763
  dimension "d56" = 1.6
  dimension "d57" = 1
  constraints: 22 point on circle, 16 end point, 14 centre point, 6 tangent, 3 collinear, 2 point on line, 1 coincident, 1 equal radius, 1 parallel, 1 perpendicular
  measures "d45" radius of A1
  measures "d46" distance from line of A0.centre L5
  measures "d47" distance of A1.centre A0.centre
  measures "d50" diameter of A13
  measures "d55" distance from line of A6.centre L5
  measures "d56" distance of A5.centre A6.centre
  measures "d57" radius of A5
extrude "Extrusion20" cut sketch "Sketch15" against normal blind 7.8994 contours L4 A9 L5 A8
extrude "Extrusion21" cut sketch "Sketch15" against normal up to surface (9.392 mm away) contours L0 A1 L7 A0
extrude "Extrusion22" add sketch "Sketch15" along normal blind 4.4958 contours A11
extrude "Extrusion23" cut sketch "Sketch15" against normal up to next contours A12
extrude "Extrusion24" cut sketch "Sketch15" against normal up to surface (9.392 mm away) contours L3 A6 L9 A5
extrude "Extrusion25" cut sketch "Sketch13" against normal up to next contours A13 | A44 A20 | A24
sketch "Sketch16" plane through (0, 0, -19.9898) normal (0, 0, -1) x (-1, 0, 0)
  arc A0 (-18.0037, 3) -> (-18.0037, -3) centre (-11.1298, 0) ccw projected
  line L0 (-18.0037, 3) -> (-18.6763, 3) projected
  line L1 (-18.6763, 3) -> (-18.6763, 8.4766) projected
  line L2 (-18.4766, 8.6763) -> (18.4766, 8.6763) projected
  line L3 (18.6763, 8.4766) -> (18.6763, -8.4766) projected
  line L4 (18.4766, -8.6763) -> (-18.4766, -8.6763) projected
  line L5 (-18.6763, -8.4766) -> (-18.6763, -3) projected
  line L6 (-18.6763, -3) -> (-18.0037, -3) projected
  line L7 (19.4765, -9.4765) -> (-19.4765, -9.4765) projected
  ellipse E0 centre (18.9997, -8.9997) end of major axis (19.7072, -9.7072) minor radius 1 (19.0003, -9.4765) -> (19.4765, -9.0003) ccw projected
  line L8 (19.4765, 9.4765) -> (19.4765, -9.4765) projected
  ellipse E1 centre (18.9997, 8.9997) end of major axis (19.7072, 9.7072) minor radius 1 (19.4765, 9.0003) -> (19.0003, 9.4765) ccw projected
  line L9 (-19.4765, 9.4765) -> (19.4765, 9.4765) projected
  ellipse E2 centre (-18.9997, 8.9997) end of major axis (-18.2921, 8.2921) minor radius 1 (-19.0003, 9.4765) -> (-19.4765, 9.0003) ccw projected
  line L10 (-19.4765, -9.4765) -> (-19.4765, 9.4765) projected
  ellipse E3 centre (-18.9997, -8.9997) end of major axis (-19.7072, -9.7072) minor radius 1 (-19.4765, -9.0003) -> (-19.0003, -9.4765) ccw projected
  point P0 (0, 0)
  constraints: 8 other
ref_plane "Work Plane4" through (-20, 0, 1.2954) normal (0, 1, 0) x (-1, 0, 0)
body "Solid1"
